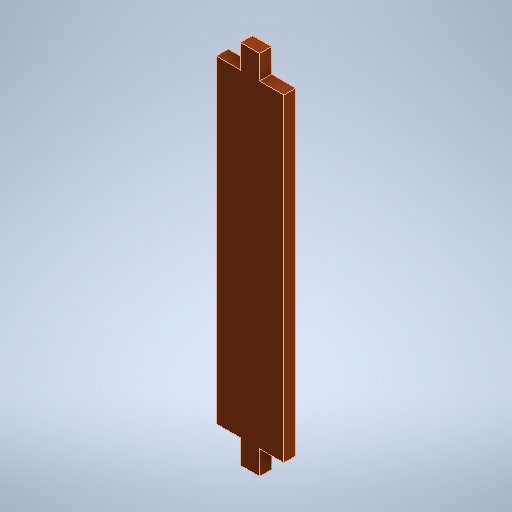
# Autodesk Inventor part: Path Holder
Saved by Autodesk Inventor 2025.4 (Build 294407000, 407)
## iProperties
Created: 2026-04-10
Part Number: Path Holder
Material: Generic
Document SubType Name: Sheet Metal
Designer: lenovo
Density: 1 g/cm^3
Sheet Metal Rule: Default_mm
Appearance: Default(1)
Author: lenovo
Autodesk Inventor part; units mm, degrees
ref_plane "YZ Plane" through (0, 0, 0) normal (1, 0, 0) x (0, 1, 0)
ref_plane "XZ Plane" through (0, 0, 0) normal (0, 1, 0) x (-1, 0, 0)
ref_plane "XY Plane" through (0, 0, 0) normal (0, 0, 1) x (1, 0, 0)
sketch "Sketch1" plane through (0, 0, 0) normal (0, 0, 1) x (1, 0, 0)
  line L0 (-8.5, -40) -> (8.5, -40)
  line L1 (8.5, -40) -> (8.5, 40)
  line L2 (8.5, 40) -> (-8.5, 40)
  line L3 (-8.5, 40) -> (-8.5, -40)
  line L4 (-8.5, -40) -> (8.5, 40) construction
  line L5 (8.5, -40) -> (-8.5, 40) construction
  line L6 (-2.4, 46) -> (2.4, 46)
  line L7 (2.4, 46) -> (2.4, 40)
  line L8 (2.4, 40) -> (-2.4, 40)
  line L9 (-2.4, 40) -> (-2.4, 46)
  line L10 (-2.4, 46) -> (2.4, 40) construction
  line L11 (2.4, 46) -> (-2.4, 40) construction
  line L12 (-8.5, 0) -> (8.5, 0)
  line L13 (-2.4, -46) -> (2.4, -46)
  line L14 (2.4, -46) -> (2.4, -40)
  line L15 (2.4, -40) -> (-2.4, -40)
  line L16 (-2.4, -40) -> (-2.4, -46)
  line L17 (-2.4, -46) -> (2.4, -40) construction
  line L18 (2.4, -46) -> (-2.4, -40) construction
  point P0 (0, 0)
  point P1 (0, 43)
  point P2 (0, 40)
  point P3 (0, 40)
  point P4 (0, -43)
  point P5 (0, -40)
  point P6 (0, -40)
  point P7 (-2.4, -40)
  point P8 (2.4, -40)
  dimension "d0" = 17
  dimension "d1" = 80
  dimension "d2" = 4.8
  dimension "d3" = 6
  measures "d0" distance of L2.end L1.end
  measures "d1" distance of L1.end L0.end
  measures "d2" distance of L7.end L8.end
  measures "d3" distance of L6.end L7.end
extrude "Plate1" add sketch "Sketch1" along normal mid plane 3
equation "\"d4\" = Thickness"
equation "\"BendRadius\" = Thickness"
equation "\"BendReliefWidth\" = Thickness"
equation "\"BendReliefDepth\" = 0.5 * Thickness"
equation "\"CornerReliefSize\" = 4 * Thickness"
equation "\"MinimumRemnant\" = 2 * Thickness"
equation "\"TransitionRadius\" = BendRadius"
equation "\"JacobiRadiusSize\" = BendRadius"
equation "\"GapSize\" = Thickness"
equation "\"Thickness\" = 3"
body "Solid1"
